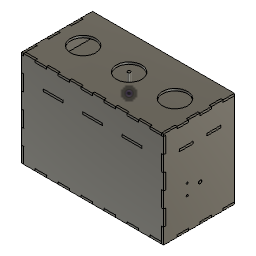
sculpture (Autodesk Fusion 360 design; units mm, degrees)
part number: 2026-07-01-00-19-11-980
part number: 2026-07-01-00-19-28-416
part number: 2026-07-01-00-26-59-999
part number: 2026-07-01-00-46-43-562
part number: 2026-07-01-01-15-33-159
part number: 2026-07-01-01-48-08-575
part number: 2026-07-01-01-53-07-553
part number: 2026-07-01-02-16-58-972
part number: 2026-07-01-02-57-53-794
part number: 2026-07-01-13-20-22-407
part number: 2026-07-01-13-51-28-464
part number: 2026-07-01-13-54-13-313
Autodesk Fusion 360 part; units mm, degrees
note: some values were not read from the file. Chosen so that the rebuilt part matches the saved one: a direction. Set by a fixed rule: which sketch regions a step uses.
(part 1 of 2)
sketch "Sketch1" plane through (0, 0, 0) normal (0, 0, 1) x (1, 0, 0) in component "BottomBox"
  line L0 (110, 55) -> (-110, 55)
  line L1 (-110, 55) -> (-110, -55) construction
  line L2 (-110, -55) -> (110, -55) construction
  line L3 (110, -55) -> (110, 55) construction
  line L4 (110, 55) -> (-110, -55) construction
  line L5 (-110, 55) -> (110, -55) construction
  line L6 (-110, -55) -> (-91.6667, -55)
  line L7 (-91.6667, -55) -> (-91.6667, -58.4)
  line L8 (-91.6667, -58.4) -> (-73.3333, -58.4)
  line L9 (-73.3333, -58.4) -> (-73.3333, -55)
  line L10 (-36.6667, -58.4) -> (-36.6667, -55)
  line L11 (-55, -58.4) -> (-36.6667, -58.4)
  line L12 (-55, -55) -> (-55, -58.4)
  line L13 (-73.3333, -55) -> (-55, -55)
  line L14 (0, -58.4) -> (0, -55)
  line L15 (-18.3333, -58.4) -> (0, -58.4)
  line L16 (-18.3333, -55) -> (-18.3333, -58.4)
  line L17 (-36.6667, -55) -> (-18.3333, -55)
  line L18 (36.6667, -58.4) -> (36.6667, -55)
  line L19 (18.3333, -58.4) -> (36.6667, -58.4)
  line L20 (18.3333, -55) -> (18.3333, -58.4)
  line L21 (0, -55) -> (18.3333, -55)
  line L22 (73.3333, -58.4) -> (73.3333, -55)
  line L23 (55, -58.4) -> (73.3333, -58.4)
  line L24 (55, -55) -> (55, -58.4)
  line L25 (36.6667, -55) -> (55, -55)
  line L26 (110, -58.4) -> (110, -55)
  line L27 (91.6667, -58.4) -> (110, -58.4)
  line L28 (91.6667, -55) -> (91.6667, -58.4)
  line L29 (73.3333, -55) -> (91.6667, -55)
  line L30 (-110, -55) -> (-110, -36.6667)
  line L31 (-110, -36.6667) -> (-113.4, -36.6667)
  line L32 (-113.4, -36.6667) -> (-113.4, -18.3333)
  line L33 (-113.4, -18.3333) -> (-110, -18.3333)
  line L34 (-110, -18.3333) -> (-110, 0)
  line L35 (-110, 0) -> (-113.4, 0)
  line L36 (-113.4, 0) -> (-113.4, 18.3333)
  line L37 (-113.4, 18.3333) -> (-110, 18.3333)
  line L38 (-110, 18.3333) -> (-110, 36.6667)
  line L39 (-110, 36.6667) -> (-113.4, 36.6667)
  line L40 (-113.4, 36.6667) -> (-113.4, 55)
  line L41 (-113.4, 55) -> (-110, 55)
  line L42 (0, 55) -> (0, -55) construction
  line L43 (113.4, 55) -> (110, 55)
  line L44 (113.4, 36.6667) -> (113.4, 55)
  line L45 (110, 36.6667) -> (113.4, 36.6667)
  line L46 (110, 18.3333) -> (110, 36.6667)
  line L47 (113.4, 18.3333) -> (110, 18.3333)
  line L48 (113.4, 0) -> (113.4, 18.3333)
  line L49 (110, 0) -> (113.4, 0)
  line L50 (110, -18.3333) -> (110, 0)
  line L51 (113.4, -18.3333) -> (110, -18.3333)
  line L52 (113.4, -36.6667) -> (113.4, -18.3333)
  line L53 (110, -36.6667) -> (113.4, -36.6667)
  line L54 (110, -55) -> (110, -36.6667)
  dimension "d7" = 220
  dimension "d8" = 110
  dimension "d9" = 18.3333
  dimension "d10" = 3.4
  dimension "d13" = 36.6667
  dimension "d14" = 0
  dimension "d15" = 18.3333
  dimension "d16" = 3.4
  dimension "d19" = 0
  dimension "d20" = 36.6667
  constraint horizontal L0
  constraint perpendicular L0 L1
  constraint parallel L0 L2
  constraint parallel L1 L3
  constraint coincident L4 origin
  constraint coincident L5 origin
  constraint perpendicular L1 L6
  constraint perpendicular L2 L7
  constraint perpendicular L7 L8
  constraint equal L6 L8
  constraint coincident L2 L9.end
  constraint perpendicular L2 L9
  constraint perpendicular L2 L30
  constraint perpendicular L30 L31
  constraint perpendicular L31 L32
  constraint equal L30 L32
  constraint coincident L1 L33.end
  constraint perpendicular L1 L33
  constraint midpoint L0 L42.start
  constraint symmetric L1.end L42 L2.end
  constraint symmetric L30.end L42 L53.start
  constraint symmetric L31.end L42 L52.start
  constraint symmetric L32.end L42 L51.start
  constraint symmetric L33.end L42 L50.start
  constraint symmetric L34.end L42 L49.start
  constraint symmetric L35.end L42 L48.start
  constraint symmetric L36.end L42 L47.start
  constraint symmetric L37.end L42 L46.start
  constraint symmetric L38.end L42 L45.start
  constraint symmetric L39.end L42 L44.start
  constraint symmetric L40.end L42 L43.start
  constraint symmetric L0.end L42 L0.start
  measures "d7" distance of L1.end L2.end
  measures "d8" distance of L0.end L1.end
  measures "d9" distance of L1.end L6.end
  measures "d10" distance of L6.end L7.end
  measures "d15" distance of L1.end L30.end
  measures "d16" distance of L30.end L31.end
extrude "Extrude1" add sketch "Sketch1" along normal blind 3.4 makes body 1 in component "BottomBox"
sketch "Sketch1 (2)" plane through (0, -58.4, 0) normal (0, -1, 0) x (1, 0, 0) in component "BackBox"
  line L0 (-91.6667, 0) -> (-73.3333, 0)
  line L1 (-73.3333, 0) -> (-73.3333, 3.4)
  line L2 (-73.3333, 3.4) -> (-91.6667, 3.4)
  line L3 (-91.6667, 3.4) -> (-91.6667, 0)
  line L4 (-110, 0) -> (-110, 3.4)
  line L5 (-110, 0) -> (-91.6667, 0)
  line L6 (-91.6667, 0) -> (-91.6667, 3.4)
  line L7 (-91.6667, 3.4) -> (-110, 3.4)
  line L8 (-110, 3.4) -> (-110, 0)
  line L9 (-73.3333, 0) -> (-55, 0)
  line L10 (-55, 0) -> (-55, 3.4)
  line L11 (-55, 3.4) -> (-73.3333, 3.4)
  line L12 (-73.3333, 3.4) -> (-73.3333, 0)
  line L13 (-55, 0) -> (-36.6667, 0)
  line L14 (-36.6667, 0) -> (-36.6667, 3.4)
  line L15 (-36.6667, 3.4) -> (-55, 3.4)
  line L16 (-55, 3.4) -> (-55, 0)
  line L17 (-36.6667, 0) -> (-18.3333, 0)
  line L18 (-18.3333, 0) -> (-18.3333, 3.4)
  line L19 (-18.3333, 3.4) -> (-36.6667, 3.4)
  line L20 (-36.6667, 3.4) -> (-36.6667, 0)
  line L21 (-18.3333, 0) -> (0, 0)
  line L22 (0, 0) -> (0, 3.4)
  line L23 (0, 3.4) -> (-18.3333, 3.4)
  line L24 (-18.3333, 3.4) -> (-18.3333, 0)
  line L25 (0, 0) -> (18.3333, 0)
  line L26 (18.3333, 0) -> (18.3333, 3.4)
  line L27 (18.3333, 3.4) -> (0, 3.4)
  line L28 (0, 3.4) -> (0, 0)
  line L29 (18.3333, 3.4) -> (36.6667, 3.4)
  line L30 (18.3333, 0) -> (36.6667, 0)
  line L31 (36.6667, 0) -> (36.6667, 3.4)
  line L32 (36.6667, 3.4) -> (18.3333, 3.4)
  line L33 (18.3333, 3.4) -> (18.3333, 0)
  line L34 (36.6667, 0) -> (55, 0)
  line L35 (55, 0) -> (55, 3.4)
  line L36 (55, 3.4) -> (36.6667, 3.4)
  line L37 (36.6667, 3.4) -> (36.6667, 0)
  line L38 (55, 0) -> (73.3333, 0)
  line L39 (73.3333, 0) -> (73.3333, 3.4)
  line L40 (73.3333, 3.4) -> (55, 3.4)
  line L41 (55, 3.4) -> (55, 0)
  line L42 (73.3333, 0) -> (91.6667, 0)
  line L43 (91.6667, 0) -> (91.6667, 3.4)
  line L44 (91.6667, 3.4) -> (73.3333, 3.4)
  line L45 (73.3333, 3.4) -> (73.3333, 0)
  line L46 (91.6667, 0) -> (110, 0)
  line L47 (110, 0) -> (110, 3.4)
  line L48 (110, 3.4) -> (91.6667, 3.4)
  line L49 (91.6667, 3.4) -> (91.6667, 0)
  line L50 (110, 3.4) -> (110, 0)
  line L51 (-110, 0) -> (110, 0)
  line L52 (110, 0) -> (110, 150) construction
  line L53 (110, 150) -> (-110, 150) construction
  line L54 (-110, 150) -> (-110, 0) construction
  line L55 (-110, 0) -> (-110, 25)
  line L56 (-110, 25) -> (-113.4, 25)
  line L57 (-113.4, 25) -> (-113.4, 50)
  line L58 (-113.4, 50) -> (-110, 50)
  line L59 (0, 150) -> (0, 0) construction
  line L60 (-110, 50) -> (-110, 75)
  line L61 (-110, 75) -> (-113.4, 75)
  line L62 (-113.4, 75) -> (-113.4, 100)
  line L63 (-113.4, 100) -> (-110, 100)
  line L64 (-110, 100) -> (-110, 125)
  line L65 (-110, 125) -> (-113.4, 125)
  line L66 (-113.4, 125) -> (-113.4, 150)
  line L67 (-113.4, 150) -> (-110, 150)
  line L68 (110, 0) -> (110, 25)
  line L69 (110, 25) -> (113.4, 25)
  line L70 (113.4, 25) -> (113.4, 50)
  line L71 (113.4, 50) -> (110, 50)
  line L72 (110, 50) -> (110, 75)
  line L73 (110, 75) -> (113.4, 75)
  line L74 (113.4, 75) -> (113.4, 100)
  line L75 (113.4, 100) -> (110, 100)
  line L76 (110, 100) -> (110, 125)
  line L77 (110, 125) -> (113.4, 125)
  line L78 (113.4, 125) -> (113.4, 150)
  line L79 (113.4, 150) -> (110, 150)
  line L80 (-78.5714, 120) -> (-47.1429, 120)
  line L81 (-47.1429, 120) -> (-47.1429, 116.6)
  line L82 (-47.1429, 116.6) -> (-78.5714, 116.6)
  line L83 (-78.5714, 116.6) -> (-78.5714, 120)
  line L84 (-15.7143, 120) -> (15.7143, 120)
  line L85 (15.7143, 116.6) -> (-15.7143, 116.6)
  line L86 (-15.7143, 116.6) -> (-15.7143, 120)
  line L87 (15.7143, 120) -> (15.7143, 116.6)
  line L88 (47.1429, 120) -> (78.5714, 120)
  line L89 (78.5714, 116.6) -> (47.1429, 116.6)
  line L90 (47.1429, 116.6) -> (47.1429, 120)
  line L91 (78.5714, 120) -> (78.5714, 116.6)
  line L92 (-110, 150) -> (-110, 153.4)
  line L93 (-110, 153.4) -> (-91.6667, 153.4)
  line L94 (-91.6667, 153.4) -> (-91.6667, 150)
  line L95 (-91.6667, 150) -> (-73.3333, 150)
  line L96 (-55, 150) -> (-36.6667, 150)
  line L97 (-55, 153.4) -> (-55, 150)
  line L98 (-73.3333, 153.4) -> (-55, 153.4)
  line L99 (-73.3333, 150) -> (-73.3333, 153.4)
  line L100 (-18.3333, 150) -> (0, 150)
  line L101 (-18.3333, 153.4) -> (-18.3333, 150)
  line L102 (-36.6667, 153.4) -> (-18.3333, 153.4)
  line L103 (-36.6667, 150) -> (-36.6667, 153.4)
  line L104 (18.3333, 150) -> (36.6667, 150)
  line L105 (18.3333, 153.4) -> (18.3333, 150)
  line L106 (0, 153.4) -> (18.3333, 153.4)
  line L107 (0, 150) -> (0, 153.4)
  line L108 (55, 150) -> (73.3333, 150)
  line L109 (55, 153.4) -> (55, 150)
  line L110 (36.6667, 153.4) -> (55, 153.4)
  line L111 (36.6667, 150) -> (36.6667, 153.4)
  line L112 (91.6667, 150) -> (110, 150)
  line L113 (91.6667, 153.4) -> (91.6667, 150)
  line L114 (73.3333, 153.4) -> (91.6667, 153.4)
  line L115 (73.3333, 150) -> (73.3333, 153.4)
  dimension "d23" = 220
  dimension "d24" = 150
  dimension "d25" = 25
  dimension "d26" = 3.4
  dimension "d29" = 0
  dimension "d30" = 50
  dimension "d51" = 30
  dimension "d52" = 31.4286
  dimension "d53" = 31.4286
  dimension "d54" = 3.4
  dimension "d76" = 125.7143
  dimension "d77" = 0
  dimension "d101" = 3.4
  dimension "d102" = 18.3333
  dimension "d105" = 36.6667
  dimension "d106" = 0
  constraint horizontal L51
  constraint vertical L52
  constraint horizontal L53
  constraint vertical L54
  constraint coincident L4.start L5.start
  constraint perpendicular L7 L55
  constraint perpendicular L54 L56
  constraint perpendicular L56 L57
  constraint equal L55 L57
  constraint coincident L54 L58.end
  constraint perpendicular L54 L58
  constraint midpoint L53 L59.start
  constraint coincident L21.end L22.start
  constraint symmetric L4.start L59 L46.end
  constraint symmetric L55.end L59 L68.end
  constraint symmetric L56.end L59 L69.end
  constraint symmetric L57.end L59 L70.end
  constraint symmetric L58.end L59 L71.end
  constraint symmetric L59 L58.end L71.end
  constraint symmetric L59 L60.end L72.end
  constraint symmetric L59 L61.end L73.end
  constraint symmetric L59 L62.end L74.end
  constraint symmetric L59 L63.end L75.end
  constraint symmetric L59 L64.end L76.end
  constraint symmetric L59 L65.end L77.end
  constraint symmetric L59 L66.end L78.end
  constraint symmetric L59 L53.end L52.end
  constraint horizontal L80
  constraint vertical L81
  constraint horizontal L82
  constraint vertical L83
  constraint perpendicular L67 L92
  constraint perpendicular L92 L93
  constraint coincident L53 L94.end
  constraint perpendicular L53 L94
  constraint coincident L53 L95.end
  constraint equal L93 L95
  measures "d23" distance of L4.start L46.end
  measures "d24" distance of L4.start L53.end
  measures "d25" distance of L4.start L55.end
  measures "d26" distance of L55.end L56.end
  measures "d51" distance of L53 L80
  measures "d52" distance of L81.end L82.end
  measures "d53" distance of L54 L83
  measures "d54" distance of L80 L82
  measures "d101" distance of L53.end L92.end
  measures "d102" distance of L92.end L93.end
extrude "Extrude1'" add sketch "Sketch1 (2)" against normal blind 3.4 separate body contours L3 L4 L5 L6 L7 L8 L51 L55 | L1 L9 L10 L11 L12 L16 L51 | L2 L7 L11 L15 L19 L23 L27 L29 L32 L36 L40 L44 L48 L55 L56 L57 L58 L60 L61 L62 L63 L64 L65 L66 L67 L68 L69 L70 L71 L72 L73 L74 L75 L76 L77 L78 L79 L92 L93 L94 L95 L96 L97 L98 L99 L100 L101 L102 L103 L104 L105 L106 L107 L108 L109 L110 L111 L112 L113 L114 L115 | L14 L17 L18 L19 L20 L24 L51 | L22 L25 L26 L27 L28 L33 L51 | L31 L34 L35 L36 L37 L41 L51 | L39 L42 L43 L44 L45 L49 L51 makes body 2 in component "BackBox"
ref_plane "WorkPlane1" through (0, 0, 76.7) normal (0, 0, 1) x (1, 0, 0)
mirror "MirrorComponent1" about plane through (0, 0, 0) normal (0, 0, 1) of bodies 1 makes body 3 in component "BottomBox(Mirror)"
sketch "Sketch1 (3)" plane through (-113.4, 0, 39.4) normal (-1, 0, 0) x (0, -1, 0) in component "BoxSide"
  line L0 (-36.6667, 114) -> (-55, 114)
  line L1 (-55, 114) -> (-55, 110.6)
  line L2 (-55, 110.6) -> (-36.6667, 110.6)
  line L3 (-36.6667, 110.6) -> (-36.6667, 114)
  line L4 (36.6667, -39.4) -> (55, -39.4)
  line L5 (55, -39.4) -> (55, -36)
  line L6 (55, -36) -> (36.6667, -36)
  line L7 (36.6667, -36) -> (36.6667, -39.4)
  line L8 (58.4, -39.4) -> (58.4, -14.4)
  line L9 (55, -14.4) -> (55, -39.4)
  line L10 (55, -39.4) -> (58.4, -39.4)
  line L11 (-55, 114) -> (58.4, 114)
  line L12 (58.4, 114) -> (58.4, -39.4)
  line L13 (58.4, -39.4) -> (-55, -39.4)
  line L14 (-55, -39.4) -> (-55, 114)
  line L15 (-33, 80.6) -> (-11, 80.6)
  line L16 (-11, 80.6) -> (-11, 77.2)
  line L17 (-11, 77.2) -> (-33, 77.2)
  line L18 (-33, 77.2) -> (-33, 80.6)
  line L19 (0, 0) -> (0, 114) construction
  line L20 (33, 80.6) -> (11, 80.6)
  line L21 (11, 77.2) -> (33, 77.2)
  line L22 (11, 80.6) -> (11, 77.2)
  line L23 (33, 77.2) -> (33, 80.6)
  line L24 (58.4, -14.4) -> (55, -14.4)
  dimension "d42" = 22
  dimension "d43" = 3.4
  dimension "d44" = 22
  dimension "d61" = 30
  constraint horizontal L11
  constraint vertical L12
  constraint horizontal L13
  constraint vertical L14
  constraint coincident L8.start L10.end
  constraint coincident L0.end L1.start
  constraint horizontal L15
  constraint vertical L16
  constraint horizontal L17
  constraint vertical L18
  constraint coincident L19.start origin
  constraint coincident L11 L19.end
  constraint perpendicular L11 L19
  constraint symmetric L15.start L19 L20.start
  constraint symmetric L15.end L19 L20.end
  constraint symmetric L16.end L19 L21.start
  constraint symmetric L17.end L19 L21.end
  measures "d42" distance of L16.end L17.end
  measures "d43" distance of L15.end L16.end
  measures "d44" distance of L14 L18
  measures "d61" distance of L2 L15
extrude "Extrude1''" add sketch "Sketch1 (3)" against normal blind 3.4 separate body makes body 4 in component "BoxSide"
combine "Combine1" operation cut target body 4 tool bodies 3 2 1 body 3 seen with x (1, 0, 0) y (0, 1, 0) z (0, 0, 1) at (0, 0, 153.4) keep tools in component "BoxSide"
mirror "MirrorComponent2" about plane through (0, 0, 0) normal (0, 0, 1) of bodies 4 makes body 5 in component "BoxSide(Mirror)"
ref_plane "WorkPlane2" through (0, 0, 120) normal (0, 0, 1) x (1, 0, 0)
sketch "Sketch3" plane through (0, 0, 120) normal (0, 0, 1) x (1, 0, 0) in component "BoxSeparator"
  line L0 (113.4, 55) -> (-113.4, 55)
  line L1 (-113.4, 55) -> (-113.4, -55)
  line L2 (113.4, -55) -> (113.4, 55)
  line L3 (113.4, 55) -> (-113.4, -55) construction
  line L4 (-113.4, 55) -> (113.4, -55) construction
  line L5 (113.4, -55) -> (-113.4, -55)
  line L6 (-113.4, -55) -> (-113.4, -58.4)
  line L7 (-113.4, -58.4) -> (113.4, -58.4)
  line L8 (113.4, -58.4) -> (113.4, -55)
  dimension "d67" = 226.8
  dimension "d68" = 110
  dimension "d69" = 3.4
  constraint horizontal L0
  constraint perpendicular L0 L1
  constraint parallel L1 L2
  constraint coincident L3 origin
  constraint coincident L4 origin
  constraint horizontal L5
  constraint vertical L6
  constraint horizontal L7
  constraint vertical L8
  constraint coincident L1.end L3.end
  measures "d67" distance of L1.end L2.start
  measures "d68" distance of L0.end L1.end
  measures "d69" distance of L1.end L6.end
extrude "Extrude2" add sketch "Sketch3" against normal blind 3.4 separate body makes body 6 in component "BoxSeparator"
combine "Combine1'" operation cut target body 6 tool bodies 5 4 2 body 5 seen with x (-1, 0, 0) y (0, 1, 0) z (0, 0, -1) at (0, 0, 0) keep tools in component "BoxSeparator"
sketch "Sketch1 (4)" plane through (-113.4, 0, 0) normal (-1, 0, 0) x (0, -1, 0)
  line L0 (36.6667, 3.4) -> (36.6667, 0)
  line L1 (36.6667, 0) -> (58.4, 0)
  line L2 (58.4, 0) -> (58.4, 25)
  line L3 (58.4, 153.4) -> (36.6667, 153.4)
  line L4 (36.6667, 153.4) -> (36.6667, 150)
  line L5 (36.6667, 150) -> (18.3333, 150)
  line L6 (18.3333, 150) -> (18.3333, 153.4)
  line L7 (18.3333, 153.4) -> (0, 153.4)
  line L8 (0, 153.4) -> (0, 150)
  line L9 (0, 150) -> (-18.3333, 150)
  line L10 (-18.3333, 150) -> (-18.3333, 153.4)
  line L11 (-18.3333, 153.4) -> (-36.6667, 153.4)
  line L12 (-36.6667, 153.4) -> (-36.6667, 150)
  line L13 (-36.6667, 150) -> (-55, 150)
  line L14 (-55, 150) -> (-55, 3.4)
  line L15 (-55, 3.4) -> (-36.6667, 3.4)
  line L16 (-36.6667, 3.4) -> (-36.6667, 0)
  line L17 (-36.6667, 0) -> (-18.3333, 0)
  line L18 (-18.3333, 0) -> (-18.3333, 3.4)
  line L19 (-18.3333, 3.4) -> (0, 3.4)
  line L20 (0, 3.4) -> (0, 0)
  line L21 (0, 0) -> (18.3333, 0)
  line L22 (18.3333, 0) -> (18.3333, 3.4)
  line L23 (18.3333, 3.4) -> (36.6667, 3.4)
  line L24 (-11, 116.6) -> (-33, 116.6)
  line L25 (-33, 116.6) -> (-33, 120)
  line L26 (-33, 120) -> (-11, 120)
  line L27 (-11, 120) -> (-11, 116.6)
  line L28 (33, 120) -> (33, 116.6)
  line L29 (33, 116.6) -> (11, 116.6)
  line L30 (11, 116.6) -> (11, 120)
  line L31 (11, 120) -> (33, 120)
  line L32 (0, 0) -> (0, 153.4) construction
  line L33 (-22, 116.6) -> (-22, 0) construction
  line L34 (-22, 58.3) -> (58.9945, 57.1955) construction
  circle A0 centre (0, 58) radius 2.4
  line L35 (58.4, 25) -> (55, 25)
  line L36 (55, 25) -> (55, 50)
  line L37 (55, 50) -> (58.4, 50)
  line L38 (58.4, 50) -> (58.4, 75)
  line L39 (58.4, 75) -> (55, 75)
  line L40 (55, 75) -> (55, 100)
  line L41 (55, 100) -> (58.4, 100)
  line L42 (58.4, 100) -> (58.4, 125)
  line L43 (58.4, 125) -> (55, 125)
  line L44 (55, 125) -> (55, 150)
  line L45 (55, 150) -> (58.4, 150)
  line L46 (58.4, 150) -> (58.4, 153.4)
  dimension "d80" = 4.8
  constraint coincident L20.end L21.start
  constraint coincident L7.end L8.start
  constraint midpoint L24 L33.start
  constraint coincident L17 L33.end
  constraint perpendicular L17 L33
  constraint midpoint L33 L34.start
  constraint coincident L32 A0.centre
  constraint coincident L34 A0.centre
  measures "d80" diameter of A0
extrude "Extrude2'" cut sketch "Sketch1 (4)" against normal blind 3.4 contours A0 bodies 4 in component "BoxSide"
sketch "Sketch2" plane through (113.4, 0, 0) normal (1, 0, 0) x (0, 1, 0)
  line L0 (-36.6667, 0) -> (-36.6667, 3.4)
  line L1 (-36.6667, 3.4) -> (-18.3333, 3.4)
  line L2 (-18.3333, 3.4) -> (-18.3333, 0)
  line L3 (-18.3333, 0) -> (0, 0)
  line L4 (0, 0) -> (0, 3.4)
  line L5 (0, 3.4) -> (18.3333, 3.4)
  line L6 (18.3333, 3.4) -> (18.3333, 0)
  line L7 (18.3333, 0) -> (36.6667, 0)
  line L8 (36.6667, 0) -> (36.6667, 3.4)
  line L9 (36.6667, 3.4) -> (55, 3.4)
  line L10 (55, 3.4) -> (55, 150)
  line L11 (55, 150) -> (36.6667, 150)
  line L12 (36.6667, 150) -> (36.6667, 153.4)
  line L13 (36.6667, 153.4) -> (18.3333, 153.4)
  line L14 (18.3333, 153.4) -> (18.3333, 150)
  line L15 (18.3333, 150) -> (0, 150)
  line L16 (0, 150) -> (0, 153.4)
  line L17 (0, 153.4) -> (-18.3333, 153.4)
  line L18 (-18.3333, 153.4) -> (-18.3333, 150)
  line L19 (-18.3333, 150) -> (-36.6667, 150)
  line L20 (-36.6667, 150) -> (-36.6667, 153.4)
  line L21 (-36.6667, 153.4) -> (-58.4, 153.4)
  line L22 (-58.4, 153.4) -> (-58.4, 150)
  line L23 (-58.4, 0) -> (-36.6667, 0)
  line L24 (33, 116.6) -> (11, 116.6)
  line L25 (11, 116.6) -> (11, 120)
  line L26 (11, 120) -> (33, 120)
  line L27 (33, 120) -> (33, 116.6)
  line L28 (-33, 116.6) -> (-33, 120)
  line L29 (-33, 120) -> (-11, 120)
  line L30 (-11, 120) -> (-11, 116.6)
  line L31 (-11, 116.6) -> (-33, 116.6)
  line L32 (0, 0) -> (0, 153.4) construction
  line L33 (-22, 116.6) -> (-22, 0) construction
  line L34 (-22, 58.3) -> (55, 58.3) construction
  circle A0 centre (0, 58.3) radius 2.7
  circle A1 centre (-20.6, 49.55) radius 1.5
  line L35 (-36.6667, 0) -> (-18.3333, 0)
  circle A2 centre (-20.6, 67.05) radius 1.5
  line L36 (-58.4, 150) -> (-55, 150)
  line L37 (-55, 150) -> (-55, 125)
  line L38 (-55, 125) -> (-58.4, 125)
  line L39 (-58.4, 125) -> (-58.4, 100)
  line L40 (-58.4, 100) -> (-55, 100)
  line L41 (-55, 100) -> (-55, 75)
  line L42 (-55, 75) -> (-58.4, 75)
  line L43 (-58.4, 75) -> (-58.4, 50)
  line L44 (-58.4, 50) -> (-55, 50)
  line L45 (-55, 50) -> (-55, 25)
  line L46 (-55, 25) -> (-58.4, 25)
  line L47 (-58.4, 25) -> (-58.4, 0)
  dimension "d83" = 5.4
  dimension "d84" = 3
  dimension "d85" = 8.75
  dimension "d86" = 20.6
  constraint coincident L3.end L4.start
  constraint coincident L16.end L17.start
  constraint midpoint L31 L33.start
  constraint perpendicular L1 L33
  constraint midpoint L33 L34.start
  constraint coincident L10 L34.end
  constraint perpendicular L10 L34
  constraint coincident L32 A0.centre
  constraint coincident L34 A0.centre
  constraint coincident L33.end L35
  constraint symmetric L34 A1 A2
  measures "d83" diameter of A0
  measures "d84" diameter of A1
  measures "d85" distance of L34 A1.centre
  measures "d86" horizontal distance of A0.centre A1.centre
extrude "Extrude1'''" cut sketch "Sketch2" against normal blind 3.4 contours A0 | A1 | A2 sketch seen with x (-1, 0, 0) y (0, 1, 0) z (0, 0, -1) at (0, 0, 0) bodies 5 in component "BoxSide(Mirror)"
sketch "Sketch1 (5)" plane through (-113.4, 0, 0) normal (-1, 0, 0) x (0, -1, 0) in component "horizontaldowel"
  circle A0 centre (0, 58) radius 2.4
  line L0 (36.6667, 3.4) -> (36.6667, 0)
  line L1 (36.6667, 0) -> (58.4, 0)
  line L2 (58.4, 0) -> (58.4, 25)
  line L3 (58.4, 153.4) -> (36.6667, 153.4)
  line L4 (36.6667, 153.4) -> (36.6667, 150)
  line L5 (36.6667, 150) -> (18.3333, 150)
  line L6 (18.3333, 150) -> (18.3333, 153.4)
  line L7 (18.3333, 153.4) -> (0, 153.4)
  line L8 (0, 153.4) -> (0, 150)
  line L9 (0, 150) -> (-18.3333, 150)
  line L10 (-18.3333, 150) -> (-18.3333, 153.4)
  line L11 (-18.3333, 153.4) -> (-36.6667, 153.4)
  line L12 (-36.6667, 153.4) -> (-36.6667, 150)
  line L13 (-36.6667, 150) -> (-55, 150)
  line L14 (-55, 150) -> (-55, 3.4)
  line L15 (-55, 3.4) -> (-36.6667, 3.4)
  line L16 (-36.6667, 3.4) -> (-36.6667, 0)
  line L17 (-36.6667, 0) -> (-18.3333, 0)
  line L18 (-18.3333, 0) -> (-18.3333, 3.4)
  line L19 (-18.3333, 3.4) -> (0, 3.4)
  line L20 (0, 3.4) -> (0, 0)
  line L21 (0, 0) -> (18.3333, 0)
  line L22 (18.3333, 0) -> (18.3333, 3.4)
  line L23 (18.3333, 3.4) -> (36.6667, 3.4)
  line L24 (-11, 116.6) -> (-33, 116.6)
  line L25 (-33, 116.6) -> (-33, 120)
  line L26 (-33, 120) -> (-11, 120)
  line L27 (-11, 120) -> (-11, 116.6)
  line L28 (33, 120) -> (33, 116.6)
  line L29 (33, 116.6) -> (11, 116.6)
  line L30 (11, 116.6) -> (11, 120)
  line L31 (11, 120) -> (33, 120)
  circle A1 centre (0, 58) radius 2.4
  line L32 (58.4, 25) -> (55, 25)
  line L33 (55, 25) -> (55, 50)
  line L34 (55, 50) -> (58.4, 50)
  line L35 (58.4, 50) -> (58.4, 75)
  line L36 (58.4, 75) -> (55, 75)
  line L37 (55, 75) -> (55, 100)
  line L38 (55, 100) -> (58.4, 100)
  line L39 (58.4, 100) -> (58.4, 125)
  line L40 (58.4, 125) -> (55, 125)
  line L41 (55, 125) -> (55, 150)
  line L42 (55, 150) -> (58.4, 150)
  line L43 (58.4, 150) -> (58.4, 153.4)
  dimension "d89" = 4.8
  constraint concentric A0 A1
  measures "d89" diameter of A1
extrude "Extrude1''''" add sketch "Sketch1 (5)" against normal blind 226.8 separate body contours A0 A1 makes body 7 in component "horizontaldowel"
sketch "Sketch1 (6)" plane through (0, 0, 0) normal (1, 0, 0) x (0, 1, 0) in component "camshaft"
  circle A0 centre (0, 58) radius 2.4
  circle A1 centre (0, 73) radius 25
  circle A2 centre (0, 58) radius 2.4
  dimension "d92" = 4.8
  dimension "d93" = 15
  dimension "d94" = 50
  constraint coincident A0.centre A2.centre
  constraint vertical A0.centre A1.centre
  measures "d92" diameter of A0
  measures "d93" vertical distance of A0.centre A1.centre
  measures "d94" diameter of A1
extrude "Extrude1'''''" add sketch "Sketch1 (6)" along normal blind 1.7 and the other way blind 1.7 separate body makes body 8 in component "camshaft"
sketch "Sketch4" plane through (0, 0, 120) normal (0, 0, 1) x (-1, 0, 0)
  line L0 (-78.5714, 55) -> (-110, 55)
  line L1 (-110, 55) -> (-110, 33)
  line L2 (-110, 33) -> (-113.4, 33)
  line L3 (-113.4, 33) -> (-113.4, 11)
  line L4 (-113.4, 11) -> (-110, 11)
  line L5 (-110, 11) -> (-110, -11)
  line L6 (-110, -11) -> (-113.4, -11)
  line L7 (-113.4, -11) -> (-113.4, -33)
  line L8 (-113.4, -33) -> (-110, -33)
  line L9 (-110, -33) -> (-110, -55)
  line L10 (-110, -55) -> (110, -55)
  line L11 (110, -55) -> (110, -33)
  line L12 (110, -33) -> (113.4, -33)
  line L13 (113.4, -33) -> (113.4, -11)
  line L14 (113.4, -11) -> (110, -11)
  line L15 (110, -11) -> (110, 11)
  line L16 (110, 11) -> (113.4, 11)
  line L17 (113.4, 11) -> (113.4, 33)
  line L18 (113.4, 33) -> (110, 33)
  line L19 (110, 33) -> (110, 55)
  line L20 (110, 55) -> (78.5714, 55)
  line L21 (78.5714, 55) -> (78.5714, 58.4)
  line L22 (78.5714, 58.4) -> (47.1429, 58.4)
  line L23 (47.1429, 58.4) -> (47.1429, 55)
  line L24 (47.1429, 55) -> (15.7143, 55)
  line L25 (15.7143, 55) -> (15.7143, 58.4)
  line L26 (15.7143, 58.4) -> (-15.7143, 58.4)
  line L27 (-15.7143, 58.4) -> (-15.7143, 55)
  line L28 (-15.7143, 55) -> (-47.1429, 55)
  line L29 (-47.1429, 55) -> (-47.1429, 58.4)
  line L30 (-47.1429, 58.4) -> (-78.5714, 58.4)
  line L31 (-78.5714, 58.4) -> (-78.5714, 55)
  circle A0 centre (0, 0) radius 2.4
  circle A1 centre (-73.3333, 0) radius 2.4
  circle A2 centre (73.3333, 0) radius 2.4
  dimension "d109" = 4.8
  dimension "d138" = 73.3333
  dimension "d139" = 0
  constraint coincident A0.centre origin
  measures "d109" diameter of A0
extrude "Extrude3" cut sketch "Sketch4" against normal blind 3.4 contours A0 | A1 | A2 bodies 6 in component "BoxSeparator"
sketch "Sketch5" plane through (0, 0, 153.4) normal (0, 0, 1) x (-1, 0, 0)
  line L0 (110, 55) -> (91.6667, 55)
  line L1 (91.6667, 55) -> (91.6667, 58.4)
  line L2 (91.6667, 58.4) -> (73.3333, 58.4)
  line L3 (73.3333, 58.4) -> (73.3333, 55)
  line L4 (73.3333, 55) -> (55, 55)
  line L5 (55, 55) -> (55, 58.4)
  line L6 (55, 58.4) -> (36.6667, 58.4)
  line L7 (36.6667, 58.4) -> (36.6667, 55)
  line L8 (36.6667, 55) -> (18.3333, 55)
  line L9 (18.3333, 55) -> (18.3333, 58.4)
  line L10 (18.3333, 58.4) -> (0, 58.4)
  line L11 (0, 58.4) -> (0, 55)
  line L12 (0, 55) -> (-18.3333, 55)
  line L13 (-18.3333, 55) -> (-18.3333, 58.4)
  line L14 (-18.3333, 58.4) -> (-36.6667, 58.4)
  line L15 (-36.6667, 58.4) -> (-36.6667, 55)
  line L16 (-36.6667, 55) -> (-55, 55)
  line L17 (-55, 55) -> (-55, 58.4)
  line L18 (-55, 58.4) -> (-73.3333, 58.4)
  line L19 (-73.3333, 58.4) -> (-73.3333, 55)
  line L20 (-73.3333, 55) -> (-91.6667, 55)
  line L21 (-91.6667, 55) -> (-91.6667, 58.4)
  line L22 (-91.6667, 58.4) -> (-110, 58.4)
  line L23 (-110, 58.4) -> (-110, 36.6667)
  line L24 (-110, 36.6667) -> (-113.4, 36.6667)
  line L25 (-113.4, 36.6667) -> (-113.4, 18.3333)
  line L26 (-113.4, 18.3333) -> (-110, 18.3333)
  line L27 (-110, 18.3333) -> (-110, 0)
  line L28 (-110, 0) -> (-113.4, 0)
  line L29 (-113.4, 0) -> (-113.4, -18.3333)
  line L30 (-113.4, -18.3333) -> (-110, -18.3333)
  line L31 (-110, -18.3333) -> (-110, -36.6667)
  line L32 (-110, -36.6667) -> (-113.4, -36.6667)
  line L33 (-113.4, -36.6667) -> (-113.4, -55)
  line L34 (-113.4, -55) -> (113.4, -55)
  line L35 (113.4, -55) -> (113.4, -36.6667)
  line L36 (113.4, -36.6667) -> (110, -36.6667)
  line L37 (110, -36.6667) -> (110, -18.3333)
  line L38 (110, -18.3333) -> (113.4, -18.3333)
  line L39 (113.4, -18.3333) -> (113.4, 0)
  line L40 (113.4, 0) -> (110, 0)
  line L41 (110, 0) -> (110, 18.3333)
  line L42 (110, 18.3333) -> (113.4, 18.3333)
  line L43 (113.4, 18.3333) -> (113.4, 36.6667)
  line L44 (113.4, 36.6667) -> (110, 36.6667)
  line L45 (110, 36.6667) -> (110, 55)
  circle A0 centre (0, 0) radius 20
  circle A1 centre (-73.3333, 0) radius 20
  circle A2 centre (73.3333, 0) radius 20
  dimension "d112" = 40
  dimension "d142" = 73.3333
  dimension "d143" = 0
  constraint coincident A0.centre origin
  measures "d112" diameter of A0
extrude "Extrude1''''''" cut sketch "Sketch5" against normal blind 3.4 contours A0 | A1 | A2 sketch seen with x (1, 0, 0) y (0, 1, 0) z (0, 0, 1) at (0, 0, -153.4) bodies 3 in component "BottomBox(Mirror)"
sketch "Sketch1 (7)" plane through (0, 0, 153.4) normal (0, 0, 1) x (-1, 0, 0) in component "dowel"
  circle A0 centre (0, 0) radius 2.4
  dimension "d115" = 4.8
  constraint coincident A0.centre origin
  measures "d115" diameter of A0
extrude "Extrude2''" add sketch "Sketch1 (7)" along normal blind 30 and the other way blind 50 separate body makes body 9 in component "dowel"
sketch "Sketch1 (8)" plane through (0, 0, 103.4) normal (0, 0, -1) x (1, 0, 0) in component "base"
  circle A0 centre (0, 0) radius 2.4
  circle A1 centre (0, 0) radius 25
  dimension "d148" = 50
  constraint coincident A0.centre A1.centre
  measures "d148" diameter of A1
extrude "Extrude1'''''''" add sketch "Sketch1 (8)" along normal blind 3.4 separate body contours A0 | A1 makes body 10 in component "base"
sketch "Sketch6" plane through (0, 0, 0) normal (0, 1, 0) x (1, 0, 0)
sketch "Sketch1 (9)" plane through (0, 0, 0) normal (0, 1, 0) x (1, 0, 0) in component "mole"
  spline S0 degree 2 poles (-22.3341, -12.6642) (-20.3525, -12.987) (-19.1998, -11.9969) knots 0 0 0 1 1 1
  spline S1 degree 2 poles (-19.1998, -11.0794) (-20.7306, -11.2414) (-21.8474, -10.1786) knots 0 0 0 1 1 1
  spline S2 degree 2 poles (-7.3401, -12.6642) (-9.3217, -12.987) (-10.4745, -11.9969) knots 0 0 0 1 1 1
  spline S3 degree 2 poles (-10.4738, -11.0794) (-8.943, -11.2414) (-7.8262, -10.1786) knots 0 0 0 1 1 1
  circle A0 centre (-18.4752, -13.9829) radius 1.1798
  circle A1 centre (-18.508, -14.4805) radius 0.4038
  circle A2 centre (-11.2138, -13.889) radius 1.1798
  circle A3 centre (-11.2466, -14.3867) radius 0.4038
  ellipse E0 centre (-14.8445, -12.3556) end of major axis (-13.8679, -12.3556) minor radius 0.7805
  spline S4 degree 2 poles (-16.5161, -11.5751) (-16.6942, -10.8987) (-15.8218, -10.7997) knots 0 0 0 1 1 1
  spline S5 degree 2 poles (-15.8218, -10.7997) (-14.975, -10.729) (-14.8451, -11.5751) knots 0 0 0 1 1 1
  spline S6 degree 2 poles (-13.1735, -11.5751) (-12.9954, -10.8987) (-13.8679, -10.7997) knots 0 0 0 1 1 1
  spline S7 degree 2 poles (-13.8679, -10.7997) (-14.7146, -10.729) (-14.8445, -11.5751) knots 0 0 0 1 1 1
  spline S8 degree 3 poles (-12.1429, -11.1797) (-12.1429, -10.214) (-13.3612, -9.4315) (-14.8638, -9.4315) knots 0 0 0 0 1 1 1 1
  spline S9 degree 3 poles (-14.8638, -9.4315) (-16.3663, -9.4315) (-17.5847, -10.214) (-17.5847, -11.1797) knots 0 0 0 0 1 1 1 1
  spline S10 degree 3 poles (-17.5847, -11.1797) (-17.5847, -11.4645) (-17.5442, -11.6966) (-17.3867, -12.0515) knots 0 0 0 0 1 1 1 1
  spline S11 degree 3 poles (-17.3867, -12.0515) (-16.8987, -13.0551) (-16.1651, -13.8035) (-14.8837, -13.8035) knots 0 0 0 0 1 1 1 1
  spline S12 degree 3 poles (-14.8837, -13.8035) (-13.6023, -13.8035) (-12.8475, -12.8031) (-12.3936, -11.9969) knots 0 0 0 0 1 1 1 1
  spline S13 degree 3 poles (-12.3936, -11.9969) (-12.193, -11.6317) (-12.1429, -11.4864) (-12.1429, -11.1797) knots 0 0 0 0 1 1 1 1
  spline S14 degree 3 poles (-19.3862, -6.9723) (-19.491, -6.6624) (-19.7025, -6.3712) (-19.9944, -6.1191) knots 0 0 0 0 1 1 1 1
  spline S15 degree 3 poles (-19.9944, -6.1191) (-19.9919, -6.2291) (-19.9976, -6.3442) (-20.0118, -6.4618) knots 0 0 0 0 1 1 1 1
  spline S16 degree 3 poles (-20.0118, -6.4618) (-20.0973, -7.1626) (-20.4625, -7.695) (-20.8277, -7.6506) knots 0 0 0 0 1 1 1 1
  spline S17 degree 3 poles (-20.8277, -7.6506) (-21.1935, -7.6062) (-21.4205, -7.0012) (-21.335, -6.3004) knots 0 0 0 0 1 1 1 1
  spline S18 degree 3 poles (-21.335, -6.3004) (-21.297, -5.9912) (-21.2051, -5.7147) (-21.0816, -5.5058) knots 0 0 0 0 1 1 1 1
  spline S19 degree 3 poles (-21.0816, -5.5058) (-21.1916, -5.4665) (-21.3054, -5.4318) (-21.4224, -5.4016) knots 0 0 0 0 1 1 1 1
  spline S20 degree 3 poles (-21.4224, -5.4016) (-21.3555, -5.6318) (-21.3337, -5.9185) (-21.371, -6.2233) knots 0 0 0 0 1 1 1 1
  spline S21 degree 3 poles (-21.371, -6.2233) (-21.4565, -6.9241) (-21.8217, -7.4564) (-22.1869, -7.4121) knots 0 0 0 0 1 1 1 1
  spline S22 degree 3 poles (-22.1869, -7.4121) (-22.5527, -7.3671) (-22.7796, -6.7627) (-22.6941, -6.0619) knots 0 0 0 0 1 1 1 1
  spline S23 degree 3 poles (-22.6941, -6.0619) (-22.6562, -5.7501) (-22.5623, -5.471) (-22.4382, -5.2621) knots 0 0 0 0 1 1 1 1
  spline S24 degree 3 poles (-22.4382, -5.2621) (-22.5424, -5.2595) (-22.6453, -5.2608) (-22.7462, -5.2666) knots 0 0 0 0 1 1 1 1
  spline S25 degree 3 poles (-22.7462, -5.2666) (-22.7083, -5.4665) (-22.7006, -5.6967) (-22.7301, -5.9385) knots 0 0 0 0 1 1 1 1
  spline S26 degree 3 poles (-22.7301, -5.9385) (-22.8156, -6.6393) (-23.1808, -7.1716) (-23.546, -7.1273) knots 0 0 0 0 1 1 1 1
  spline S27 degree 3 poles (-23.546, -7.1273) (-23.9112, -7.0822) (-24.1382, -6.4779) (-24.0533, -5.7771) knots 0 0 0 0 1 1 1 1
  spline S28 degree 3 poles (-24.0533, -5.7771) (-24.0443, -5.7012) (-24.0314, -5.6273) (-24.016, -5.5559) knots 0 0 0 0 1 1 1 1
  spline S29 degree 3 poles (-24.016, -5.5559) (-24.6493, -5.8382) (-25.082, -6.3049) (-25.1502, -6.8739) knots 0 0 0 0 1 1 1 1
  spline S30 degree 3 poles (-25.1502, -6.8739) (-25.2453, -7.6615) (-24.6152, -8.4241) (-23.6309, -8.8478) knots 0 0 0 0 1 1 1 1
  spline S31 degree 3 poles (-23.6309, -8.8478) (-23.2824, -8.9976) (-22.8889, -9.1049) (-22.4672, -9.1557) knots 0 0 0 0 1 1 1 1
  spline S32 degree 3 poles (-22.4672, -9.1557) (-20.8573, -9.3486) (-19.4486, -8.6407) (-19.32, -7.5741) knots 0 0 0 0 1 1 1 1
  spline S33 degree 3 poles (-19.32, -7.5741) (-19.2956, -7.3696) (-19.32, -7.1678) (-19.3862, -6.9723) knots 0 0 0 0 1 1 1 1
  spline S34 degree 3 poles (-22.7462, -5.2666) (-22.8176, -4.8866) (-22.9976, -4.6172) (-23.2368, -4.5883) knots 0 0 0 0 1 1 1 1
  spline S35 degree 3 poles (-23.2368, -4.5883) (-23.5627, -4.5484) (-23.8887, -4.9676) (-24.016, -5.5559) knots 0 0 0 0 1 1 1 1
  spline S36 degree 3 poles (-24.016, -5.5559) (-24.0314, -5.6273) (-24.0443, -5.7012) (-24.0533, -5.7771) knots 0 0 0 0 1 1 1 1
  spline S37 degree 3 poles (-24.0533, -5.7771) (-24.1382, -6.4779) (-23.9112, -7.0822) (-23.546, -7.1273) knots 0 0 0 0 1 1 1 1
  spline S38 degree 3 poles (-23.546, -7.1273) (-23.1808, -7.1716) (-22.8156, -6.6393) (-22.7301, -5.9385) knots 0 0 0 0 1 1 1 1
  spline S39 degree 3 poles (-22.7301, -5.9385) (-22.7006, -5.6967) (-22.7083, -5.4665) (-22.7462, -5.2666) knots 0 0 0 0 1 1 1 1
  spline S40 degree 3 poles (-21.4224, -5.4016) (-21.5092, -5.102) (-21.6712, -4.8982) (-21.8776, -4.8731) knots 0 0 0 0 1 1 1 1
  spline S41 degree 3 poles (-21.8776, -4.8731) (-22.0808, -4.8487) (-22.2833, -5.0011) (-22.4382, -5.2621) knots 0 0 0 0 1 1 1 1
  spline S42 degree 3 poles (-22.4382, -5.2621) (-22.5623, -5.471) (-22.6562, -5.7501) (-22.6941, -6.0619) knots 0 0 0 0 1 1 1 1
  spline S43 degree 3 poles (-22.6941, -6.0619) (-22.7796, -6.7627) (-22.5527, -7.3671) (-22.1869, -7.4121) knots 0 0 0 0 1 1 1 1
  spline S44 degree 3 poles (-22.1869, -7.4121) (-21.8217, -7.4564) (-21.4565, -6.9241) (-21.371, -6.2233) knots 0 0 0 0 1 1 1 1
  spline S45 degree 3 poles (-21.371, -6.2233) (-21.3337, -5.9185) (-21.3555, -5.6318) (-21.4224, -5.4016) knots 0 0 0 0 1 1 1 1
  spline S46 degree 3 poles (-19.9944, -6.1191) (-20.006, -5.5733) (-20.2143, -5.1483) (-20.5184, -5.1116) knots 0 0 0 0 1 1 1 1
  spline S47 degree 3 poles (-20.5184, -5.1116) (-20.7229, -5.0866) (-20.9267, -5.2422) (-21.0816, -5.5058) knots 0 0 0 0 1 1 1 1
  spline S48 degree 3 poles (-21.0816, -5.5058) (-21.2051, -5.7147) (-21.297, -5.9912) (-21.335, -6.3004) knots 0 0 0 0 1 1 1 1
  spline S49 degree 3 poles (-21.335, -6.3004) (-21.4205, -7.0012) (-21.1935, -7.6062) (-20.8277, -7.6506) knots 0 0 0 0 1 1 1 1
  spline S50 degree 3 poles (-20.8277, -7.6506) (-20.4625, -7.695) (-20.0973, -7.1626) (-20.0118, -6.4618) knots 0 0 0 0 1 1 1 1
  spline S51 degree 3 poles (-20.0118, -6.4618) (-19.9976, -6.3442) (-19.9919, -6.2291) (-19.9944, -6.1191) knots 0 0 0 0 1 1 1 1
  spline S52 degree 3 poles (-4.6347, -6.8739) (-4.7028, -6.3049) (-5.1355, -5.8382) (-5.7688, -5.5559) knots 0 0 0 0 1 1 1 1
  spline S53 degree 3 poles (-5.7688, -5.5559) (-5.7534, -5.6273) (-5.7405, -5.7012) (-5.7315, -5.7771) knots 0 0 0 0 1 1 1 1
  spline S54 degree 3 poles (-5.7315, -5.7771) (-5.6563, -6.4001) (-5.8273, -6.9472) (-6.1231, -7.0919) knots 0 0 0 0 1 1 1 1
  spline S55 degree 3 poles (-6.1231, -7.0919) (-6.1597, -7.1105) (-6.1983, -7.1221) (-6.2388, -7.1273) knots 0 0 0 0 1 1 1 1
  spline S56 degree 3 poles (-6.2388, -7.1273) (-6.3693, -7.1433) (-6.4992, -7.0855) (-6.6168, -6.9723) knots 0 0 0 0 1 1 1 1
  spline S57 degree 3 poles (-6.6168, -6.9723) (-6.829, -6.7698) (-6.9994, -6.3892) (-7.0547, -5.9385) knots 0 0 0 0 1 1 1 1
  spline S58 degree 3 poles (-7.0547, -5.9385) (-7.0842, -5.6967) (-7.0765, -5.4665) (-7.0386, -5.2666) knots 0 0 0 0 1 1 1 1
  spline S59 degree 3 poles (-7.0386, -5.2666) (-7.1395, -5.2608) (-7.2424, -5.2595) (-7.3466, -5.2621) knots 0 0 0 0 1 1 1 1
  spline S60 degree 3 poles (-7.3466, -5.2621) (-7.2225, -5.471) (-7.1286, -5.7501) (-7.0907, -6.0619) knots 0 0 0 0 1 1 1 1
  spline S61 degree 3 poles (-7.0907, -6.0619) (-7.0482, -6.4072) (-7.0823, -6.7293) (-7.171, -6.9723) knots 0 0 0 0 1 1 1 1
  spline S62 degree 3 poles (-7.171, -6.9723) (-7.2623, -7.2224) (-7.4121, -7.3896) (-7.598, -7.4121) knots 0 0 0 0 1 1 1 1
  spline S63 degree 3 poles (-7.598, -7.4121) (-7.8133, -7.4384) (-8.0287, -7.2636) (-8.1862, -6.9723) knots 0 0 0 0 1 1 1 1
  spline S64 degree 3 poles (-8.1862, -6.9723) (-8.2968, -6.7698) (-8.3785, -6.5107) (-8.4138, -6.2233) knots 0 0 0 0 1 1 1 1
  spline S65 degree 3 poles (-8.4138, -6.2233) (-8.4511, -5.9185) (-8.4293, -5.6318) (-8.3624, -5.4016) knots 0 0 0 0 1 1 1 1
  spline S66 degree 3 poles (-8.3624, -5.4016) (-8.4794, -5.4318) (-8.5932, -5.4665) (-8.7032, -5.5058) knots 0 0 0 0 1 1 1 1
  spline S67 degree 3 poles (-8.7032, -5.5058) (-8.5797, -5.7147) (-8.4878, -5.9912) (-8.4498, -6.3004) knots 0 0 0 0 1 1 1 1
  spline S68 degree 3 poles (-8.4498, -6.3004) (-8.4203, -6.5422) (-8.428, -6.7723) (-8.4659, -6.9723) knots 0 0 0 0 1 1 1 1
  spline S69 degree 3 poles (-8.4659, -6.9723) (-8.5373, -7.3516) (-8.7173, -7.6217) (-8.9571, -7.6506) knots 0 0 0 0 1 1 1 1
  spline S70 degree 3 poles (-8.9571, -7.6506) (-9.2265, -7.6834) (-9.4953, -7.4031) (-9.6521, -6.9723) knots 0 0 0 0 1 1 1 1
  spline S71 degree 3 poles (-9.6521, -6.9723) (-9.7087, -6.8186) (-9.7505, -6.6463) (-9.773, -6.4618) knots 0 0 0 0 1 1 1 1
  spline S72 degree 3 poles (-9.773, -6.4618) (-9.7872, -6.3442) (-9.7929, -6.2291) (-9.7904, -6.1191) knots 0 0 0 0 1 1 1 1
  spline S73 degree 3 poles (-9.7904, -6.1191) (-10.0823, -6.3712) (-10.2938, -6.6624) (-10.3986, -6.9723) knots 0 0 0 0 1 1 1 1
  spline S74 degree 3 poles (-10.3986, -6.9723) (-10.4648, -7.1678) (-10.4892, -7.3696) (-10.4648, -7.5741) knots 0 0 0 0 1 1 1 1
  spline S75 degree 3 poles (-10.4648, -7.5741) (-10.3362, -8.6407) (-8.9276, -9.3486) (-7.3176, -9.1557) knots 0 0 0 0 1 1 1 1
  spline S76 degree 3 poles (-7.3176, -9.1557) (-6.8959, -9.1049) (-6.5024, -8.9976) (-6.1539, -8.8478) knots 0 0 0 0 1 1 1 1
  spline S77 degree 3 poles (-6.1539, -8.8478) (-6.1436, -8.8433) (-6.1333, -8.8388) (-6.1231, -8.8342) knots 0 0 0 0 1 1 1 1
  spline S78 degree 3 poles (-6.1231, -8.8342) (-5.1561, -8.408) (-4.5408, -7.6532) (-4.6347, -6.8739) knots 0 0 0 0 1 1 1 1
  spline S79 degree 3 poles (-5.7315, -5.7771) (-5.7405, -5.7012) (-5.7534, -5.6273) (-5.7688, -5.5559) knots 0 0 0 0 1 1 1 1
  spline S80 degree 3 poles (-5.7688, -5.5559) (-5.8961, -4.9676) (-6.2221, -4.5484) (-6.548, -4.5883) knots 0 0 0 0 1 1 1 1
  spline S81 degree 3 poles (-6.548, -4.5883) (-6.7872, -4.6172) (-6.9672, -4.8866) (-7.0386, -5.2666) knots 0 0 0 0 1 1 1 1
  spline S82 degree 3 poles (-7.0386, -5.2666) (-7.0765, -5.4665) (-7.0842, -5.6967) (-7.0547, -5.9385) knots 0 0 0 0 1 1 1 1
  spline S83 degree 3 poles (-7.0547, -5.9385) (-6.9994, -6.3892) (-6.829, -6.7698) (-6.6168, -6.9723) knots 0 0 0 0 1 1 1 1
  spline S84 degree 3 poles (-6.6168, -6.9723) (-6.4992, -7.0855) (-6.3693, -7.1433) (-6.2388, -7.1273) knots 0 0 0 0 1 1 1 1
  spline S85 degree 3 poles (-6.2388, -7.1273) (-6.1983, -7.1221) (-6.1597, -7.1105) (-6.1231, -7.0919) knots 0 0 0 0 1 1 1 1
  spline S86 degree 3 poles (-6.1231, -7.0919) (-5.8273, -6.9472) (-5.6563, -6.4001) (-5.7315, -5.7771) knots 0 0 0 0 1 1 1 1
  spline S87 degree 3 poles (-7.0907, -6.0619) (-7.1286, -5.7501) (-7.2225, -5.471) (-7.3466, -5.2621) knots 0 0 0 0 1 1 1 1
  spline S88 degree 3 poles (-7.3466, -5.2621) (-7.5015, -5.0011) (-7.704, -4.8487) (-7.9072, -4.8731) knots 0 0 0 0 1 1 1 1
  spline S89 degree 3 poles (-7.9072, -4.8731) (-8.1136, -4.8982) (-8.2756, -5.102) (-8.3624, -5.4016) knots 0 0 0 0 1 1 1 1
  spline S90 degree 3 poles (-8.3624, -5.4016) (-8.4293, -5.6318) (-8.4511, -5.9185) (-8.4138, -6.2233) knots 0 0 0 0 1 1 1 1
  spline S91 degree 3 poles (-8.4138, -6.2233) (-8.3785, -6.5107) (-8.2968, -6.7698) (-8.1862, -6.9723) knots 0 0 0 0 1 1 1 1
  spline S92 degree 3 poles (-8.1862, -6.9723) (-8.0287, -7.2636) (-7.8133, -7.4384) (-7.598, -7.4121) knots 0 0 0 0 1 1 1 1
  spline S93 degree 3 poles (-7.598, -7.4121) (-7.4121, -7.3896) (-7.2623, -7.2224) (-7.171, -6.9723) knots 0 0 0 0 1 1 1 1
  spline S94 degree 3 poles (-7.171, -6.9723) (-7.0823, -6.7293) (-7.0482, -6.4072) (-7.0907, -6.0619) knots 0 0 0 0 1 1 1 1
  spline S95 degree 3 poles (-8.4498, -6.3004) (-8.4878, -5.9912) (-8.5797, -5.7147) (-8.7032, -5.5058) knots 0 0 0 0 1 1 1 1
  spline S96 degree 3 poles (-8.7032, -5.5058) (-8.8581, -5.2422) (-9.0619, -5.0866) (-9.2664, -5.1116) knots 0 0 0 0 1 1 1 1
  spline S97 degree 3 poles (-9.2664, -5.1116) (-9.5705, -5.1483) (-9.7788, -5.5733) (-9.7904, -6.1191) knots 0 0 0 0 1 1 1 1
  spline S98 degree 3 poles (-9.7904, -6.1191) (-9.7929, -6.2291) (-9.7872, -6.3442) (-9.773, -6.4618) knots 0 0 0 0 1 1 1 1
  spline S99 degree 3 poles (-9.773, -6.4618) (-9.7505, -6.6463) (-9.7087, -6.8186) (-9.6521, -6.9723) knots 0 0 0 0 1 1 1 1
  spline S100 degree 3 poles (-9.6521, -6.9723) (-9.4953, -7.4031) (-9.2265, -7.6834) (-8.9571, -7.6506) knots 0 0 0 0 1 1 1 1
  spline S101 degree 3 poles (-8.9571, -7.6506) (-8.7173, -7.6217) (-8.5373, -7.3516) (-8.4659, -6.9723) knots 0 0 0 0 1 1 1 1
  spline S102 degree 3 poles (-8.4659, -6.9723) (-8.428, -6.7723) (-8.4203, -6.5422) (-8.4498, -6.3004) knots 0 0 0 0 1 1 1 1
  spline S103 degree 2 poles (-6.0909, -11.5909) (-3.2813, -12.5977) (-2.7766, -10.1513) knots 0 0 0 1 1 1
  spline S104 degree 2 poles (-2.7766, -10.1513) (-0.291, -9.3952) (-2.0198, -6.9456) knots 0 0 0 1 1 1
  spline S105 degree 2 poles (-2.0198, -6.9456) (-0.867, -4.316) (-3.5327, -4.1354) knots 0 0 0 1 1 1
  spline S106 degree 2 poles (-3.5327, -4.1354) (-4.1454, -3.4513) (-5.0461, -3.5953) knots 0 0 0 1 1 1
  spline S107 degree 2 poles (-5.0461, -3.5953) (-6.1989, -1.6498) (-8.3997, -2.6225) knots 0 0 0 1 1 1
  spline S108 degree 2 poles (-8.3997, -2.6225) (-9.6644, -1.2177) (-11.2138, -1.9018) knots 0 0 0 1 1 1
  spline S109 degree 2 poles (-11.2138, -1.9018) (-11.9783, -1.5058) (-13.1259, -2.0458) knots 0 0 0 1 1 1
  spline S110 degree 2 poles (-13.1259, -2.0458) (-14.9744, -1.001) (-16.4988, -2.0818) knots 0 0 0 1 1 1
  spline S111 degree 2 poles (-16.4988, -2.0818) (-17.5763, -1.3257) (-18.443, -1.9378) knots 0 0 0 1 1 1
  spline S112 degree 2 poles (-18.443, -1.9378) (-20.204, -1.2897) (-21.3208, -2.6225) knots 0 0 0 1 1 1
  spline S113 degree 2 poles (-21.3208, -2.6225) (-24.1221, -1.6498) (-24.5715, -3.6313) knots 0 0 0 1 1 1
  spline S114 degree 2 poles (-24.5715, -3.6313) (-25.6876, -3.5593) (-26.2284, -4.0634) knots 0 0 0 1 1 1
  spline S115 degree 2 poles (-26.2284, -4.0634) (-29.182, -4.9641) (-27.5972, -7.1032) knots 0 0 0 1 1 1
  spline S116 degree 2 poles (-27.5972, -7.1032) (-29.7587, -9.4582) (-26.7324, -10.4188) knots 0 0 0 1 1 1
  spline S117 degree 2 poles (-26.7324, -10.4188) (-25.5076, -12.7385) (-23.5987, -11.5484) knots 0 0 0 1 1 1
  line L0 (-6.0909, -12.1087) -> (-6.0909, -8.8703)
  spline S118 degree 3 poles (-6.0909, -8.8703) (-6.1012, -8.8748) (-6.1115, -8.8793) (-6.1218, -8.8838) knots 0 0 0 0 1 1 1 1
  spline S119 degree 3 poles (-6.1218, -8.8838) (-6.4702, -9.0336) (-6.8637, -9.1409) (-7.2855, -9.1917) knots 0 0 0 0 1 1 1 1
  spline S120 degree 3 poles (-7.2855, -9.1917) (-8.8954, -9.3846) (-10.3041, -8.6767) (-10.4327, -7.6101) knots 0 0 0 0 1 1 1 1
  spline S121 degree 3 poles (-10.4327, -7.6101) (-10.4571, -7.4056) (-10.4648, -7.1678) (-10.3986, -6.9723) knots 0 0 0 0 1 1 1 1
  line L1 (-10.3986, -6.9723) -> (-10.6808, -6.9948)
  spline S122 degree 3 poles (-10.6808, -6.9948) (-11.1129, -6.9588) (-11.2576, -6.6393) (-11.3495, -6.2991) knots 0 0 0 0 1 1 1 1
  spline S123 degree 2 poles (-11.3495, -6.2991) (-11.6054, -6.7646) (-11.9976, -7.0077) knots 0 0 0 1 1 1
  spline S124 degree 3 poles (-11.9976, -7.0077) (-12.2541, -7.1678) (-12.5692, -7.2321) (-12.9093, -7.0077) knots 0 0 0 0 1 1 1 1
  spline S125 degree 3 poles (-12.9093, -7.0077) (-13.1041, -6.8784) (-13.3066, -6.6547) (-13.5111, -6.2991) knots 0 0 0 0 1 1 1 1
  spline S126 degree 2 poles (-13.5111, -6.2991) (-13.8383, -6.7691) (-14.3237, -7.0077) knots 0 0 0 1 1 1
  spline S127 degree 3 poles (-14.3237, -7.0077) (-14.6291, -7.1575) (-14.9969, -7.2153) (-15.3859, -7.0077) knots 0 0 0 0 1 1 1 1
  spline S128 degree 3 poles (-15.3859, -7.0077) (-15.6205, -6.8816) (-15.8636, -6.6586) (-16.1047, -6.2991) knots 0 0 0 0 1 1 1 1
  spline S129 degree 2 poles (-16.1047, -6.2991) (-16.3181, -6.7293) (-16.6602, -7.0077) knots 0 0 0 1 1 1
  spline S130 degree 3 poles (-16.6602, -7.0077) (-16.9578, -7.2501) (-17.3532, -7.378) (-17.7911, -7.0077) knots 0 0 0 0 1 1 1 1
  spline S131 degree 3 poles (-17.7911, -7.0077) (-17.9454, -6.8771) (-18.1042, -6.6856) (-18.2662, -6.4162) knots 0 0 0 0 1 1 1 1
  spline S132 degree 2 poles (-18.2662, -6.4162) (-18.3106, -6.5943) (-18.4353, -6.7871) knots 0 0 0 1 1 1
  spline S133 degree 3 poles (-18.4353, -6.7871) (-18.5253, -6.9267) (-18.6841, -7.0077) (-18.85, -7.0077) knots 0 0 0 0 1 1 1 1
  line L2 (-18.85, -7.0077) -> (-19.3534, -7.0077)
  spline S134 degree 3 poles (-19.3534, -7.0077) (-19.2872, -7.2031) (-19.2628, -7.405) (-19.2872, -7.6095) knots 0 0 0 0 1 1 1 1
  spline S135 degree 3 poles (-19.2872, -7.6095) (-19.4158, -8.6761) (-20.8245, -9.384) (-22.4344, -9.1911) knots 0 0 0 0 1 1 1 1
  spline S136 degree 3 poles (-22.4344, -9.1911) (-22.8562, -9.1403) (-23.2496, -9.0329) (-23.5981, -8.8831) knots 0 0 0 0 1 1 1 1
  line L3 (-23.5981, -8.8831) -> (-23.5981, -12.1081)
  spline S137 degree 3 poles (-23.5981, -12.1081) (-23.5987, -17.7074) (-19.6788, -22.2466) (-14.8445, -22.2466) knots 0 0 0 0 1 1 1 1
  spline S138 degree 3 poles (-14.8445, -22.2466) (-10.0103, -22.2466) (-6.0909, -17.7074) (-6.0909, -12.1087) knots 0 0 0 0 1 1 1 1
  point P0 (-17.2954, -13.9829)
  point P1 (-18.1042, -14.4805)
  point P2 (-10.034, -13.889)
  point P3 (-10.8429, -14.3867)
  point P4 (-13.8679, -12.3556)
  point P5 (-6.0909, -11.5909)
  point P6 (-23.5987, -11.5484)
  constraint coincident L0 P5
  constraint coincident P5 S103.start
  constraint coincident P6 S117.end
sketch "Sketch1 (10)" plane through (0, 0, 0) normal (0, 0, 1) x (1, 0, 0) in component "Shaft Holder"
  circle A0 centre (0, 0) radius 2.7
  line L0 (1.85, 3) -> (-1.85, 3)
  line L1 (-1.85, 3) -> (-1.85, -3)
  line L2 (-1.85, -3) -> (1.85, -3)
  line L3 (1.85, -3) -> (1.85, 3)
  line L4 (1.85, 3) -> (-1.85, -3) construction
  line L5 (-1.85, 3) -> (1.85, -3) construction
  circle A1 centre (0, 0) radius 7.5
  dimension "d170" = 5.4
  dimension "d171" = 3.7
  dimension "d172" = 6
  dimension "d173" = 15
  constraint coincident A0.centre A1.centre
  constraint horizontal L0
  constraint perpendicular L0 L1
  constraint parallel L0 L2
  constraint parallel L1 L3
  constraint coincident L4 A0.centre
  constraint coincident L5 A0.centre
  measures "d170" diameter of A0
  measures "d171" distance of L1.end L2.end
  measures "d172" distance of L0.end L1.end
  measures "d173" diameter of A1
extrude "Extrude1''''''''" add sketch "Sketch1 (10)" along normal blind 3.4 separate body contours A0 L3 | A0 L0 L1 L3 | A0 L1 L2 L3 | A0 L1 | A1 makes body 11 in component "Shaft Holder"
sketch "Sketch1 (11)" plane through (0, 0, 0) normal (0, 0, 1) x (1, 0, 0) in component "dowel holder"
  circle A0 centre (0, 0) radius 2.4
  circle A1 centre (0, 0) radius 7.5
  dimension "d176" = 4.8
  dimension "d177" = 15
  constraint coincident A0.centre A1.centre
  constraint concentric A0 A1
  measures "d176" diameter of A0
  measures "d177" diameter of A1
extrude "Extrude1'''''''''" add sketch "Sketch1 (11)" along normal blind 3.4 separate body makes body 12 in component "dowel holder"